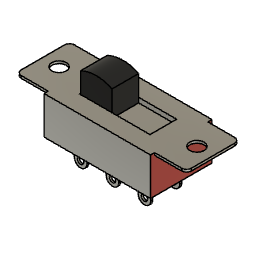
ELT Slide Switch v16 (Autodesk Fusion 360 archive; units mm, degrees)
design "Slide Switch DP3T"
Autodesk Fusion 360 part; units mm, degrees
sketch "Sketch1" plane through (0, 0, 0) normal (0, 0, 1) x (1, 0, 0) in component "Metal"
  line L0 (0, 6.35) -> (11, 6.35)
  line L1 (11, 6.35) -> (11, 5.5)
  line L2 (11, 5.5) -> (16.6, 5.5)
  line L3 (17.6, 4.5) -> (17.6, 0)
  line L4 (0, 0) -> (0, 6.35) construction
  line L5 (17.6, 0) -> (0, 0) construction
  arc A0 (17.6, 4.5) -> (16.6, 5.5) centre (16.6, 4.5) ccw
  line L6 (0, -6.35) -> (11, -6.35)
  line L7 (11, -6.35) -> (11, -5.5)
  line L8 (11, -5.5) -> (16.6, -5.5)
  arc A1 (16.6, -5.5) -> (17.6, -4.5) centre (16.6, -4.5) ccw
  line L9 (17.6, -4.5) -> (17.6, 0)
  line L10 (0, 6.35) -> (-11, 6.35)
  line L11 (-11, 6.35) -> (-11, 5.5)
  line L12 (-11, 5.5) -> (-16.6, 5.5)
  arc A2 (-16.6, 5.5) -> (-17.6, 4.5) centre (-16.6, 4.5) ccw
  line L13 (-17.6, 4.5) -> (-17.6, 0)
  line L14 (0, -6.35) -> (-11, -6.35)
  line L15 (-11, -6.35) -> (-11, -5.5)
  line L16 (-11, -5.5) -> (-16.6, -5.5)
  arc A3 (-17.6, -4.5) -> (-16.6, -5.5) centre (-16.6, -4.5) ccw
  line L17 (-17.6, -4.5) -> (-17.6, 0)
  line L18 (7.3, 2.75) -> (-7.3, 2.75)
  line L19 (-7.3, 2.75) -> (-7.3, -2.75)
  line L20 (-7.3, -2.75) -> (7.3, -2.75)
  line L21 (7.3, -2.75) -> (7.3, 2.75)
  line L22 (7.3, 2.75) -> (-7.3, -2.75) construction
  line L23 (-7.3, 2.75) -> (7.3, -2.75) construction
  circle A4 centre (14.25, 0) radius 1.5
  circle A5 centre (-14.25, 0) radius 1.5
  line L24 (11, 5.5) -> (11, -5.5)
  line L25 (-11, 5.5) -> (-11, -5.5)
  point P0 (17.6, 5.5)
  dimension "d1" = 5.5
  dimension "d2" = 6.35
  dimension "d3" = 11
  dimension "d4" = 17.6
  dimension "d5" = 1
  dimension "d6" = 14.6
  dimension "d7" = 5.5
  dimension "d8" = 3
  dimension "d9" = 14.25
  constraint horizontal L0
  constraint perpendicular L0 L1
  constraint perpendicular L1 L2
  constraint perpendicular L2 L3
  constraint horizontal L4.start L3.end
  constraint vertical L4.start L0.start
  constraint coincident L4.start L5.end
  constraint coincident P0 L2
  constraint coincident P0 L3
  constraint tangent L2 A0
  constraint tangent L3 A0
  constraint symmetric L0.start L5 L6.start
  constraint symmetric L0.end L5 L6.end
  constraint symmetric L1.end L5 L7.end
  constraint symmetric L3.end L5 L9.end
  constraint symmetric L5 L2.end L8.end
  constraint symmetric L5 L3.start A1.end
  constraint symmetric L5 A0 A1
  constraint symmetric L0.start L4 L10.start
  constraint symmetric L0.end L4 L10.end
  constraint symmetric L1.end L4 L11.end
  constraint symmetric L3.end L4 L13.end
  constraint symmetric L4 L2.end L12.end
  constraint symmetric L4 L3.start A2.end
  constraint symmetric L4 A0 A2
  constraint symmetric L4 L6.start L14.start
  constraint symmetric L4 L6.end L14.end
  constraint symmetric L4 L7.end L15.end
  constraint symmetric L4 L8.end L16.end
  constraint symmetric L4 A1.end A3.start
  constraint symmetric L4 A1 A3
  constraint symmetric L4 L3.end L13.end
  constraint horizontal L18
  constraint perpendicular L18 L19
  constraint parallel L18 L20
  constraint parallel L19 L21
  constraint coincident L22 L4.start
  constraint coincident L23 L4.start
  constraint coincident L5 A4.centre
  constraint symmetric L4 A4 A5
  measures "d1" distance of P0 L3.end
  measures "d2" distance of L4.start L0
  measures "d3" distance of L0.start L0.end
  measures "d4" distance of L4.start L3
  measures "d5" radius of A0
  measures "d6" distance of L19.end L20.end
  measures "d7" distance of L18.end L19.end
  measures "d8" diameter of A4
  measures "d9" distance of L4.start A4.centre
extrude "Extrude1" add sketch "Sketch1" against normal blind 0.5 makes body 1 in component "Metal"
extrude "Extrude2" add sketch "Sketch1" against normal blind 7.8 contours L0 L1 L6 L7 L10 L11 L14 L15 L24 L25 | L18 L19 L20 L21 bodies 1 in component "Metal"
ref_plane "WorkPlane1" through (0, -3, 0) normal (0, 1, 0) x (0, 0, 1) in component "Metal"
sketch "Sketch2" plane through (0, -3, 0) normal (0, 1, 0) x (1, 0, 0) in component "Metal"
  line L0 (1.3, 7.8) -> (1.3, 11.4)
  arc A0 (1.3, 11.4) -> (-1.3, 11.4) centre (0, 11.4) ccw
  line L1 (-1.3, 11.4) -> (-1.3, 7.8)
  arc A1 (-1.3, 7.8) -> (1.3, 7.8) centre (0, 7.8) ccw
  line L2 (0, 7.8) -> (0, 11.4) construction
  line L3 (11, 7.8) -> (-11, 7.8)
  circle A2 centre (0, 11.4) radius 0.65
  circle A3 centre (-6.6, 11.4) radius 0.65
  line L4 (-6.6, 7.8) -> (-6.6, 11.4) construction
  arc A4 (-5.3, 11.4) -> (-7.9, 11.4) centre (-6.6, 11.4) ccw
  line L5 (-5.3, 7.8) -> (-5.3, 11.4)
  line L6 (-7.9, 11.4) -> (-7.9, 7.8)
  circle A5 centre (6.6, 11.4) radius 0.65
  line L7 (6.6, 7.8) -> (6.6, 11.4) construction
  arc A6 (7.9, 11.4) -> (5.3, 11.4) centre (6.6, 11.4) ccw
  line L8 (7.9, 7.8) -> (7.9, 11.4)
  line L9 (5.3, 11.4) -> (5.3, 7.8)
  dimension "d15" = 1.3
  dimension "d16" = 12.7
  dimension "d17" = 1.3
  dimension "d20" = 6.6
  dimension "d21" = 0
  constraint tangent L0 A0
  constraint tangent A0 L1
  constraint parallel L0 L1
  constraint tangent L1 A1
  constraint tangent L0 A1
  constraint vertical A1.centre origin
  constraint midpoint A1.centre L3
  constraint concentric A0 A2
  measures "d15" radius of A0
  measures "d17" diameter of A2
extrude "Extrude3" add sketch "Sketch2" along normal mid plane 0.4 contours L0 A0 L1 L3 | L3 A6 L8 L9 | L3 A4 L5 L6 bodies 1 in component "Metal"
mirror "Mirror1" about plane through (0, 0, 0) normal (0, 1, 0) of "Extrude3" in component "Metal"
extrude "Extrude4" cut sketch "Sketch1" against normal blind 1 contours L18 L19 L20 L21 bodies 1 in component "Metal"
sketch "Sketch1 (2)" plane through (0, 0, 0) normal (0, 1, 0) x (1, 0, 0) in component "Switch"
  line L0 (-7.05, -4.25) -> (-0.55, -4.25) construction
  line L1 (-0.55, -4.25) -> (-0.55, 1)
  line L2 (-0.55, 1) -> (-7.05, 1)
  line L3 (-7.05, 1) -> (-7.05, -4.25)
  arc A0 (-7.05, -4.25) -> (-0.55, -4.25) centre (-3.8, 2.4167) ccw
  line L4 (-11, 0) -> (11, 0)
  line L5 (7.3, 1) -> (-7.3, 1)
  dimension "d28" = 5
  dimension "d29" = 0.25
  dimension "d30" = 4.25
  dimension "d31" = 6.5
  constraint horizontal L0
  constraint vertical L1
  constraint horizontal L2
  constraint vertical L3
  constraint coincident L2.end L5
  measures "d28" distance of A0 L4
  measures "d29" distance of L2.end L5.end
  measures "d30" vertical distance of origin L0.start
  measures "d31" distance of L0.start L0.end
extrude "Extrude1'" add sketch "Sketch1 (2)" along normal mid plane 5.5 separate body makes body 2 in component "Switch"
component "Metal" placed x (1, 0, 0) y (0, 1, 0) z (0, 0, 1) at (0, 0, 0)
component "Switch" placed x (1, 0, 0) y (0, 1, 0) z (0, 0, 1) at (0, 0, 0)
equation "d1 = ( 11 / 2 ) * 1 mm"
equation "d2 = ( 12.7 / 2 ) * 1 mm"
equation "d4 = ( 35.2 / 2 ) * 1 mm"
equation "d6 = 6.5 mm + 2.7 mm + 2.7 mm + 2.7 mm"
equation "d9 = ( 28.5 / 2 ) * 1 mm"
equation "d15 = 2.6 mm / 2"
equation "d30 = d28 - 0.75 mm"
